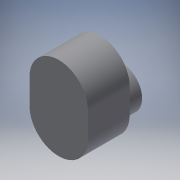
# Autodesk Inventor part: pomp
Saved by Autodesk Inventor 2017 (Build 210142000, 142)
## iProperties
Created: 2017-02-22
Part Number: pomp
Material: Generic
Document SubType Name: Modeling
Designer: user
Density: 1 g/cm^3
Appearance: Default
Author: user
Autodesk Inventor part; units mm, degrees
ref_plane "YZ Plane" through (0, 0, 0) normal (1, 0, 0) x (0, 1, 0)
ref_plane "XZ Plane" through (0, 0, 0) normal (0, 1, 0) x (-1, 0, 0)
ref_plane "XY Plane" through (0, 0, 0) normal (0, 0, 1) x (1, 0, 0)
sketch "Sketch1" plane through (0, 0, 0) normal (0, 1, 0) x (-1, 0, 0)
  line L0 (70, 30) -> (70, -30)
  arc A0 (-70, -30) -> (70, -30) centre (0, -30) ccw
  line L1 (-70, -30) -> (-70, 30)
  arc A1 (70, 30) -> (-70, 30) centre (0, 30) ccw
  point P0 (0, 0)
  point P1 (70, 0)
  dimension "d0" = 60
  dimension "d1" = 70
  constraints: 4 end point, 4 point on circle, 4 tangent, 3 horizontal alignment, 2 centre point, 2 vertical alignment, 1 midpoint, 1 parallel, 1 vertical
  measures "d0" distance of A1.centre A0.centre
  measures "d1" radius of A1
extrude "Extrusion1" add sketch "Sketch1" along normal blind 100
sketch "Sketch2" plane through (0, 100, 0) normal (0, 1, 0) x (1, 0, 0)
  line L0 (-70, 30) -> (-70, -30) projected
  arc A0 (-70, -30) -> (70, -30) centre (0, -30) ccw projected
  line L1 (70, -30) -> (70, 30) projected
  arc A1 (70, 30) -> (-70, 30) centre (0, 30) ccw projected
  circle A2 centre (0, 30) radius 50
  point P0 (0, 0)
  dimension "d4" = 100
  constraints: 1 centre point, 1 coincident
  measures "d4" diameter of A2
extrude "Extrusion2" add sketch "Sketch2" along normal blind 50 contours A2
body "Solid1"
